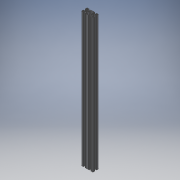
# Autodesk Inventor part: PERFIL_ESTRUTURAL_30X60_640MM
Saved by Autodesk Inventor 2018 (Build 220112000, 112)
## iProperties
Created: 2018-10-10
Part Number: PERFIL_ESTRUTURAL_30X60_640MM
Material: Genérico
Document SubType Name: Modeling
Designer: Georgines
Density: 1 g/cm^3
Appearance: Padrão
Author: Georgines
Autodesk Inventor part; units mm, degrees
ref_plane "YZ Plane" through (0, 0, 0) normal (1, 0, 0) x (0, 1, 0)
ref_plane "XZ Plane" through (0, 0, 0) normal (0, 1, 0) x (-1, 0, 0)
ref_plane "XY Plane" through (0, 0, 0) normal (0, 0, 1) x (1, 0, 0)
sketch "Esboço1" plane through (0, 0, 0) normal (0, 0, 1) x (1, 0, 0)
  arc A0 (-7.8, -13) -> (-7.5, -12.7) centre (-7.8, -12.7) ccw
  line L0 (-10.95, -13) -> (-7.8, -13)
  line L1 (-10.95, -15) -> (-10.95, -13)
  line L2 (-8.4, -15) -> (-10.95, -15)
  line L3 (-8.4, -14.7) -> (-8.4, -15)
  line L4 (-6.2, -14.7) -> (-8.4, -14.7)
  line L5 (-6.2, -15) -> (-6.2, -14.7)
  line L6 (6.2, -15) -> (-6.2, -15)
  line L7 (6.2, -14.7) -> (6.2, -15)
  line L8 (8.4, -14.7) -> (6.2, -14.7)
  line L9 (8.4, -15) -> (8.4, -14.7)
  line L10 (10.95, -15) -> (8.4, -15)
  line L11 (10.95, -13) -> (10.95, -15)
  line L12 (7.8, -13) -> (10.95, -13)
  arc A1 (7.5, -12.7) -> (7.8, -13) centre (7.8, -12.7) ccw
  line L13 (7.5, -11.9376) -> (7.5, -12.7)
  arc A2 (7.5879, -11.7255) -> (7.5, -11.9376) centre (7.8, -11.9376) ccw
  line L14 (10.779, -8.5343) -> (7.5879, -11.7255)
  arc A3 (11.3447, -8.3) -> (10.779, -8.5343) centre (11.3447, -9.1) ccw
  line L15 (18.6553, -8.3) -> (11.3447, -8.3)
  arc A4 (19.221, -8.5343) -> (18.6553, -8.3) centre (18.6553, -9.1) ccw
  line L16 (22.4121, -11.7255) -> (19.221, -8.5343)
  arc A5 (22.5, -11.9376) -> (22.4121, -11.7255) centre (22.2, -11.9376) ccw
  line L17 (22.5, -12.7) -> (22.5, -11.9376)
  arc A6 (22.2, -13) -> (22.5, -12.7) centre (22.2, -12.7) ccw
  line L18 (19.05, -13) -> (22.2, -13)
  line L19 (19.05, -15) -> (19.05, -13)
  line L20 (21.6, -15) -> (19.05, -15)
  line L21 (21.6, -14.7) -> (21.6, -15)
  line L22 (23.8, -14.7) -> (21.6, -14.7)
  line L23 (23.8, -15) -> (23.8, -14.7)
  line L24 (28.5, -15) -> (23.8, -15)
  arc A7 (28.5, -15) -> (30, -13.5) centre (28.5, -13.5) ccw
  line L25 (30, -8.8) -> (30, -13.5)
  line L26 (29.7, -8.8) -> (30, -8.8)
  line L27 (29.7, -6.6) -> (29.7, -8.8)
  line L28 (30, -6.6) -> (29.7, -6.6)
  line L29 (30, -4.05) -> (30, -6.6)
  line L30 (28, -4.05) -> (30, -4.05)
  line L31 (28, -7.2) -> (28, -4.05)
  arc A8 (27.7, -7.5) -> (28, -7.2) centre (27.7, -7.2) ccw
  line L32 (26.9376, -7.5) -> (27.7, -7.5)
  arc A9 (26.7255, -7.4121) -> (26.9376, -7.5) centre (26.9376, -7.2) ccw
  line L33 (23.5343, -4.221) -> (26.7255, -7.4121)
  arc A10 (23.3, -3.6553) -> (23.5343, -4.221) centre (24.1, -3.6553) ccw
  line L34 (23.3, 3.6553) -> (23.3, -3.6553)
  arc A11 (23.5343, 4.221) -> (23.3, 3.6553) centre (24.1, 3.6553) ccw
  line L35 (26.7255, 7.4121) -> (23.5343, 4.221)
  arc A12 (26.9376, 7.5) -> (26.7255, 7.4121) centre (26.9376, 7.2) ccw
  line L36 (27.7, 7.5) -> (26.9376, 7.5)
  arc A13 (28, 7.2) -> (27.7, 7.5) centre (27.7, 7.2) ccw
  line L37 (28, 4.05) -> (28, 7.2)
  line L38 (30, 4.05) -> (28, 4.05)
  line L39 (30, 6.6) -> (30, 4.05)
  line L40 (29.7, 6.6) -> (30, 6.6)
  line L41 (29.7, 8.8) -> (29.7, 6.6)
  line L42 (30, 8.8) -> (29.7, 8.8)
  line L43 (30, 13.5) -> (30, 8.8)
  arc A14 (30, 13.5) -> (28.5, 15) centre (28.5, 13.5) ccw
  line L44 (23.8, 15) -> (28.5, 15)
  line L45 (23.8, 14.7) -> (23.8, 15)
  line L46 (21.6, 14.7) -> (23.8, 14.7)
  line L47 (21.6, 15) -> (21.6, 14.7)
  line L48 (19.05, 15) -> (21.6, 15)
  line L49 (19.05, 13) -> (19.05, 15)
  line L50 (22.2, 13) -> (19.05, 13)
  arc A15 (22.5, 12.7) -> (22.2, 13) centre (22.2, 12.7) ccw
  line L51 (22.5, 11.9376) -> (22.5, 12.7)
  arc A16 (22.4121, 11.7255) -> (22.5, 11.9376) centre (22.2, 11.9376) ccw
  line L52 (19.221, 8.5343) -> (22.4121, 11.7255)
  arc A17 (18.6553, 8.3) -> (19.221, 8.5343) centre (18.6553, 9.1) ccw
  line L53 (11.3447, 8.3) -> (18.6553, 8.3)
  arc A18 (10.779, 8.5343) -> (11.3447, 8.3) centre (11.3447, 9.1) ccw
  line L54 (7.5879, 11.7255) -> (10.779, 8.5343)
  arc A19 (7.5, 11.9376) -> (7.5879, 11.7255) centre (7.8, 11.9376) ccw
  line L55 (7.5, 12.7) -> (7.5, 11.9376)
  arc A20 (7.8, 13) -> (7.5, 12.7) centre (7.8, 12.7) ccw
  line L56 (10.95, 13) -> (7.8, 13)
  line L57 (10.95, 15) -> (10.95, 13)
  line L58 (8.4, 15) -> (10.95, 15)
  line L59 (8.4, 14.7) -> (8.4, 15)
  line L60 (6.2, 14.7) -> (8.4, 14.7)
  line L61 (6.2, 15) -> (6.2, 14.7)
  line L62 (-6.2, 15) -> (6.2, 15)
  line L63 (-6.2, 14.7) -> (-6.2, 15)
  line L64 (-8.4, 14.7) -> (-6.2, 14.7)
  line L65 (-8.4, 15) -> (-8.4, 14.7)
  line L66 (-10.95, 15) -> (-8.4, 15)
  line L67 (-10.95, 13) -> (-10.95, 15)
  line L68 (-7.8, 13) -> (-10.95, 13)
  arc A21 (-7.5, 12.7) -> (-7.8, 13) centre (-7.8, 12.7) ccw
  line L69 (-7.5, 11.9376) -> (-7.5, 12.7)
  arc A22 (-7.5879, 11.7255) -> (-7.5, 11.9376) centre (-7.8, 11.9376) ccw
  line L70 (-10.779, 8.5343) -> (-7.5879, 11.7255)
  arc A23 (-11.3447, 8.3) -> (-10.779, 8.5343) centre (-11.3447, 9.1) ccw
  line L71 (-18.6553, 8.3) -> (-11.3447, 8.3)
  arc A24 (-19.221, 8.5343) -> (-18.6553, 8.3) centre (-18.6553, 9.1) ccw
  line L72 (-22.4121, 11.7255) -> (-19.221, 8.5343)
  arc A25 (-22.5, 11.9376) -> (-22.4121, 11.7255) centre (-22.2, 11.9376) ccw
  line L73 (-22.5, 12.7) -> (-22.5, 11.9376)
  arc A26 (-22.2, 13) -> (-22.5, 12.7) centre (-22.2, 12.7) ccw
  line L74 (-19.05, 13) -> (-22.2, 13)
  line L75 (-19.05, 15) -> (-19.05, 13)
  line L76 (-21.6, 15) -> (-19.05, 15)
  line L77 (-21.6, 14.7) -> (-21.6, 15)
  line L78 (-23.8, 14.7) -> (-21.6, 14.7)
  line L79 (-23.8, 15) -> (-23.8, 14.7)
  line L80 (-28.5, 15) -> (-23.8, 15)
  arc A27 (-28.5, 15) -> (-30, 13.5) centre (-28.5, 13.5) ccw
  line L81 (-30, 8.8) -> (-30, 13.5)
  line L82 (-29.7, 8.8) -> (-30, 8.8)
  line L83 (-29.7, 6.6) -> (-29.7, 8.8)
  line L84 (-30, 6.6) -> (-29.7, 6.6)
  line L85 (-30, 4.05) -> (-30, 6.6)
  line L86 (-28, 4.05) -> (-30, 4.05)
  line L87 (-28, 7.2) -> (-28, 4.05)
  arc A28 (-27.7, 7.5) -> (-28, 7.2) centre (-27.7, 7.2) ccw
  line L88 (-26.9376, 7.5) -> (-27.7, 7.5)
  arc A29 (-26.7255, 7.4121) -> (-26.9376, 7.5) centre (-26.9376, 7.2) ccw
  line L89 (-23.5343, 4.221) -> (-26.7255, 7.4121)
  arc A30 (-23.3, 3.6553) -> (-23.5343, 4.221) centre (-24.1, 3.6553) ccw
  line L90 (-23.3, -3.6553) -> (-23.3, 3.6553)
  arc A31 (-23.5343, -4.221) -> (-23.3, -3.6553) centre (-24.1, -3.6553) ccw
  line L91 (-26.7255, -7.4121) -> (-23.5343, -4.221)
  arc A32 (-26.9376, -7.5) -> (-26.7255, -7.4121) centre (-26.9376, -7.2) ccw
  line L92 (-27.7, -7.5) -> (-26.9376, -7.5)
  arc A33 (-28, -7.2) -> (-27.7, -7.5) centre (-27.7, -7.2) ccw
  line L93 (-28, -4.05) -> (-28, -7.2)
  line L94 (-30, -4.05) -> (-28, -4.05)
  line L95 (-30, -6.6) -> (-30, -4.05)
  line L96 (-29.7, -6.6) -> (-30, -6.6)
  line L97 (-29.7, -8.8) -> (-29.7, -6.6)
  line L98 (-30, -8.8) -> (-29.7, -8.8)
  line L99 (-30, -13.5) -> (-30, -8.8)
  arc A34 (-30, -13.5) -> (-28.5, -15) centre (-28.5, -13.5) ccw
  line L100 (-23.8, -15) -> (-28.5, -15)
  line L101 (-23.8, -14.7) -> (-23.8, -15)
  line L102 (-21.6, -14.7) -> (-23.8, -14.7)
  line L103 (-21.6, -15) -> (-21.6, -14.7)
  line L104 (-19.05, -15) -> (-21.6, -15)
  line L105 (-19.05, -13) -> (-19.05, -15)
  line L106 (-22.2, -13) -> (-19.05, -13)
  arc A35 (-22.5, -12.7) -> (-22.2, -13) centre (-22.2, -12.7) ccw
  line L107 (-22.5, -11.9376) -> (-22.5, -12.7)
  arc A36 (-22.4121, -11.7255) -> (-22.5, -11.9376) centre (-22.2, -11.9376) ccw
  line L108 (-19.221, -8.5343) -> (-22.4121, -11.7255)
  arc A37 (-18.6553, -8.3) -> (-19.221, -8.5343) centre (-18.6553, -9.1) ccw
  line L109 (-11.3447, -8.3) -> (-18.6553, -8.3)
  arc A38 (-10.779, -8.5343) -> (-11.3447, -8.3) centre (-11.3447, -9.1) ccw
  line L110 (-7.5879, -11.7255) -> (-10.779, -8.5343)
  arc A39 (-7.5, -11.9376) -> (-7.5879, -11.7255) centre (-7.8, -11.9376) ccw
  line L111 (-7.5, -12.7) -> (-7.5, -11.9376)
  arc A40 (21.0258, -8.0765) -> (21.0258, -8.5007) centre (21.238, -8.2886) ccw
  line L112 (21.0258, -8.0765) -> (23.0765, -6.0258)
  arc A41 (23.5007, -6.0258) -> (23.0765, -6.0258) centre (23.2886, -6.238) ccw
  line L113 (23.5007, -6.0258) -> (26.187, -8.7121)
  arc A42 (26.187, -8.7121) -> (26.3991, -8.8) centre (26.3991, -8.5) ccw
  line L114 (26.3991, -8.8) -> (28.4, -8.8)
  arc A43 (28.7, -9.1) -> (28.4, -8.8) centre (28.4, -9.1) ccw
  line L115 (28.7, -9.1) -> (28.7, -13.4)
  arc A44 (28.4, -13.7) -> (28.7, -13.4) centre (28.4, -13.4) ccw
  line L116 (28.4, -13.7) -> (24.1, -13.7)
  arc A45 (23.8, -13.4) -> (24.1, -13.7) centre (24.1, -13.4) ccw
  line L117 (23.8, -13.4) -> (23.8, -11.3991)
  arc A46 (23.8, -11.3991) -> (23.7121, -11.187) centre (23.5, -11.3991) ccw
  line L118 (23.7121, -11.187) -> (21.0258, -8.5007)
  arc A47 (9.57, 2.6678) -> (9.5129, 3.0123) centre (9.3007, 2.8001) ccw
  line L119 (9.5129, 3.0123) -> (7.8428, 4.6823)
  arc A48 (7.8428, 5.1066) -> (7.8428, 4.6823) centre (8.0549, 4.8945) ccw
  line L120 (7.8428, 5.1066) -> (9.8934, 7.1572)
  arc A49 (10.3177, 7.1572) -> (9.8934, 7.1572) centre (10.1055, 6.9451) ccw
  line L121 (10.3177, 7.1572) -> (11.9877, 5.4871)
  arc A50 (11.9877, 5.4871) -> (12.3322, 5.43) centre (12.1999, 5.6993) ccw
  arc A51 (13.5232, 5.867) -> (12.3322, 5.43) centre (15, 0) ccw
  arc A52 (13.5232, 5.867) -> (13.75, 6.1579) centre (13.45, 6.1579) ccw
  line L122 (13.75, 6.1579) -> (13.75, 6.7)
  arc A53 (14.05, 7) -> (13.75, 6.7) centre (14.05, 6.7) ccw
  line L123 (14.05, 7) -> (15.95, 7)
  arc A54 (16.25, 6.7) -> (15.95, 7) centre (15.95, 6.7) ccw
  line L124 (16.25, 6.7) -> (16.25, 6.1579)
  arc A55 (16.25, 6.1579) -> (16.4768, 5.867) centre (16.55, 6.1579) ccw
  arc A56 (17.6678, 5.43) -> (16.4768, 5.867) centre (15, 0) ccw
  arc A57 (17.6678, 5.43) -> (18.0123, 5.4871) centre (17.8001, 5.6993) ccw
  line L125 (18.0123, 5.4871) -> (19.6823, 7.1572)
  arc A58 (20.1066, 7.1572) -> (19.6823, 7.1572) centre (19.8945, 6.9451) ccw
  line L126 (20.1066, 7.1572) -> (22.1572, 5.1066)
  arc A59 (22.1572, 4.6823) -> (22.1572, 5.1066) centre (21.9451, 4.8945) ccw
  line L127 (22.1572, 4.6823) -> (20.4871, 3.0123)
  arc A60 (20.4871, 3.0123) -> (20.43, 2.6678) centre (20.6993, 2.8001) ccw
  arc A61 (20.867, 1.4768) -> (20.43, 2.6678) centre (15, 0) ccw
  arc A62 (20.867, 1.4768) -> (21.1579, 1.25) centre (21.1579, 1.55) ccw
  line L128 (21.1579, 1.25) -> (21.7, 1.25)
  arc A63 (22, 0.95) -> (21.7, 1.25) centre (21.7, 0.95) ccw
  line L129 (22, 0.95) -> (22, -0.95)
  arc A64 (21.7, -1.25) -> (22, -0.95) centre (21.7, -0.95) ccw
  line L130 (21.7, -1.25) -> (21.1579, -1.25)
  arc A65 (21.1579, -1.25) -> (20.867, -1.4768) centre (21.1579, -1.55) ccw
  arc A66 (20.43, -2.6678) -> (20.867, -1.4768) centre (15, 0) ccw
  arc A67 (20.43, -2.6678) -> (20.4871, -3.0123) centre (20.6993, -2.8001) ccw
  line L131 (20.4871, -3.0123) -> (22.1572, -4.6823)
  arc A68 (22.1572, -5.1066) -> (22.1572, -4.6823) centre (21.9451, -4.8945) ccw
  line L132 (22.1572, -5.1066) -> (20.1066, -7.1572)
  arc A69 (19.6823, -7.1572) -> (20.1066, -7.1572) centre (19.8945, -6.9451) ccw
  line L133 (19.6823, -7.1572) -> (18.0123, -5.4871)
  arc A70 (18.0123, -5.4871) -> (17.6678, -5.43) centre (17.8001, -5.6993) ccw
  arc A71 (16.4768, -5.867) -> (17.6678, -5.43) centre (15, 0) ccw
  arc A72 (16.4768, -5.867) -> (16.25, -6.1579) centre (16.55, -6.1579) ccw
  line L134 (16.25, -6.1579) -> (16.25, -6.7)
  arc A73 (15.95, -7) -> (16.25, -6.7) centre (15.95, -6.7) ccw
  line L135 (15.95, -7) -> (14.05, -7)
  arc A74 (13.75, -6.7) -> (14.05, -7) centre (14.05, -6.7) ccw
  line L136 (13.75, -6.7) -> (13.75, -6.1579)
  arc A75 (13.75, -6.1579) -> (13.5232, -5.867) centre (13.45, -6.1579) ccw
  arc A76 (12.3322, -5.43) -> (13.5232, -5.867) centre (15, 0) ccw
  arc A77 (12.3322, -5.43) -> (11.9877, -5.4871) centre (12.1999, -5.6993) ccw
  line L137 (11.9877, -5.4871) -> (10.3177, -7.1572)
  arc A78 (9.8934, -7.1572) -> (10.3177, -7.1572) centre (10.1055, -6.9451) ccw
  line L138 (9.8934, -7.1572) -> (7.8428, -5.1066)
  arc A79 (7.8428, -4.6823) -> (7.8428, -5.1066) centre (8.0549, -4.8945) ccw
  line L139 (7.8428, -4.6823) -> (9.5129, -3.0123)
  arc A80 (9.5129, -3.0123) -> (9.57, -2.6678) centre (9.3007, -2.8001) ccw
  arc A81 (9.133, -1.4768) -> (9.57, -2.6678) centre (15, 0) ccw
  arc A82 (9.133, -1.4768) -> (8.8421, -1.25) centre (8.8421, -1.55) ccw
  line L140 (8.8421, -1.25) -> (8.3, -1.25)
  arc A83 (8, -0.95) -> (8.3, -1.25) centre (8.3, -0.95) ccw
  line L141 (8, -0.95) -> (8, 0.95)
  arc A84 (8.3, 1.25) -> (8, 0.95) centre (8.3, 0.95) ccw
  line L142 (8.3, 1.25) -> (8.8421, 1.25)
  arc A85 (8.8421, 1.25) -> (9.133, 1.4768) centre (8.8421, 1.55) ccw
  arc A86 (9.57, 2.6678) -> (9.133, 1.4768) centre (15, 0) ccw
  arc A87 (-9.133, 1.4768) -> (-9.57, 2.6678) centre (-15, 0) ccw
  arc A88 (-9.133, 1.4768) -> (-8.8421, 1.25) centre (-8.8421, 1.55) ccw
  line L143 (-8.8421, 1.25) -> (-8.3, 1.25)
  arc A89 (-8, 0.95) -> (-8.3, 1.25) centre (-8.3, 0.95) ccw
  line L144 (-8, 0.95) -> (-8, -0.95)
  arc A90 (-8.3, -1.25) -> (-8, -0.95) centre (-8.3, -0.95) ccw
  line L145 (-8.3, -1.25) -> (-8.8421, -1.25)
  arc A91 (-8.8421, -1.25) -> (-9.133, -1.4768) centre (-8.8421, -1.55) ccw
  arc A92 (-9.57, -2.6678) -> (-9.133, -1.4768) centre (-15, 0) ccw
  arc A93 (-9.57, -2.6678) -> (-9.5129, -3.0123) centre (-9.3007, -2.8001) ccw
  line L146 (-9.5129, -3.0123) -> (-7.8428, -4.6823)
  arc A94 (-7.8428, -5.1066) -> (-7.8428, -4.6823) centre (-8.0549, -4.8945) ccw
  line L147 (-7.8428, -5.1066) -> (-9.8934, -7.1572)
  arc A95 (-10.3177, -7.1572) -> (-9.8934, -7.1572) centre (-10.1055, -6.9451) ccw
  line L148 (-10.3177, -7.1572) -> (-11.9877, -5.4871)
  arc A96 (-11.9877, -5.4871) -> (-12.3322, -5.43) centre (-12.1999, -5.6993) ccw
  arc A97 (-13.5232, -5.867) -> (-12.3322, -5.43) centre (-15, 0) ccw
  arc A98 (-13.5232, -5.867) -> (-13.75, -6.1579) centre (-13.45, -6.1579) ccw
  line L149 (-13.75, -6.1579) -> (-13.75, -6.7)
  arc A99 (-14.05, -7) -> (-13.75, -6.7) centre (-14.05, -6.7) ccw
  line L150 (-14.05, -7) -> (-15.95, -7)
  arc A100 (-16.25, -6.7) -> (-15.95, -7) centre (-15.95, -6.7) ccw
  line L151 (-16.25, -6.7) -> (-16.25, -6.1579)
  arc A101 (-16.25, -6.1579) -> (-16.4768, -5.867) centre (-16.55, -6.1579) ccw
  arc A102 (-17.6678, -5.43) -> (-16.4768, -5.867) centre (-15, 0) ccw
  arc A103 (-17.6678, -5.43) -> (-18.0123, -5.4871) centre (-17.8001, -5.6993) ccw
  line L152 (-18.0123, -5.4871) -> (-19.6823, -7.1572)
  arc A104 (-20.1066, -7.1572) -> (-19.6823, -7.1572) centre (-19.8945, -6.9451) ccw
  line L153 (-20.1066, -7.1572) -> (-22.1572, -5.1066)
  arc A105 (-22.1572, -4.6823) -> (-22.1572, -5.1066) centre (-21.9451, -4.8945) ccw
  line L154 (-22.1572, -4.6823) -> (-20.4871, -3.0123)
  arc A106 (-20.4871, -3.0123) -> (-20.43, -2.6678) centre (-20.6993, -2.8001) ccw
  arc A107 (-20.867, -1.4768) -> (-20.43, -2.6678) centre (-15, 0) ccw
  arc A108 (-20.867, -1.4768) -> (-21.1579, -1.25) centre (-21.1579, -1.55) ccw
  line L155 (-21.1579, -1.25) -> (-21.7, -1.25)
  arc A109 (-22, -0.95) -> (-21.7, -1.25) centre (-21.7, -0.95) ccw
  line L156 (-22, -0.95) -> (-22, 0.95)
  arc A110 (-21.7, 1.25) -> (-22, 0.95) centre (-21.7, 0.95) ccw
  line L157 (-21.7, 1.25) -> (-21.1579, 1.25)
  arc A111 (-21.1579, 1.25) -> (-20.867, 1.4768) centre (-21.1579, 1.55) ccw
  arc A112 (-20.43, 2.6678) -> (-20.867, 1.4768) centre (-15, 0) ccw
  arc A113 (-20.43, 2.6678) -> (-20.4871, 3.0123) centre (-20.6993, 2.8001) ccw
  line L158 (-20.4871, 3.0123) -> (-22.1572, 4.6823)
  arc A114 (-22.1572, 5.1066) -> (-22.1572, 4.6823) centre (-21.9451, 4.8945) ccw
  line L159 (-22.1572, 5.1066) -> (-20.1066, 7.1572)
  arc A115 (-19.6823, 7.1572) -> (-20.1066, 7.1572) centre (-19.8945, 6.9451) ccw
  line L160 (-19.6823, 7.1572) -> (-18.0123, 5.4871)
  arc A116 (-18.0123, 5.4871) -> (-17.6678, 5.43) centre (-17.8001, 5.6993) ccw
  arc A117 (-16.4768, 5.867) -> (-17.6678, 5.43) centre (-15, 0) ccw
  arc A118 (-16.4768, 5.867) -> (-16.25, 6.1579) centre (-16.55, 6.1579) ccw
  line L161 (-16.25, 6.1579) -> (-16.25, 6.7)
  arc A119 (-15.95, 7) -> (-16.25, 6.7) centre (-15.95, 6.7) ccw
  line L162 (-15.95, 7) -> (-14.05, 7)
  arc A120 (-13.75, 6.7) -> (-14.05, 7) centre (-14.05, 6.7) ccw
  line L163 (-13.75, 6.7) -> (-13.75, 6.1579)
  arc A121 (-13.75, 6.1579) -> (-13.5232, 5.867) centre (-13.45, 6.1579) ccw
  arc A122 (-12.3322, 5.43) -> (-13.5232, 5.867) centre (-15, 0) ccw
  arc A123 (-12.3322, 5.43) -> (-11.9877, 5.4871) centre (-12.1999, 5.6993) ccw
  line L164 (-11.9877, 5.4871) -> (-10.3177, 7.1572)
  arc A124 (-9.8934, 7.1572) -> (-10.3177, 7.1572) centre (-10.1055, 6.9451) ccw
  line L165 (-9.8934, 7.1572) -> (-7.8428, 5.1066)
  arc A125 (-7.8428, 4.6823) -> (-7.8428, 5.1066) centre (-8.0549, 4.8945) ccw
  line L166 (-7.8428, 4.6823) -> (-9.5129, 3.0123)
  arc A126 (-9.5129, 3.0123) -> (-9.57, 2.6678) centre (-9.3007, 2.8001) ccw
  arc A127 (26.3991, 8.8) -> (26.187, 8.7121) centre (26.3991, 8.5) ccw
  line L167 (26.187, 8.7121) -> (23.5007, 6.0258)
  arc A128 (23.0765, 6.0258) -> (23.5007, 6.0258) centre (23.2886, 6.238) ccw
  line L168 (23.0765, 6.0258) -> (21.0258, 8.0765)
  arc A129 (21.0258, 8.5007) -> (21.0258, 8.0765) centre (21.238, 8.2886) ccw
  line L169 (21.0258, 8.5007) -> (23.7121, 11.187)
  arc A130 (23.7121, 11.187) -> (23.8, 11.3991) centre (23.5, 11.3991) ccw
  line L170 (23.8, 11.3991) -> (23.8, 13.4)
  arc A131 (24.1, 13.7) -> (23.8, 13.4) centre (24.1, 13.4) ccw
  line L171 (24.1, 13.7) -> (28.4, 13.7)
  arc A132 (28.7, 13.4) -> (28.4, 13.7) centre (28.4, 13.4) ccw
  line L172 (28.7, 13.4) -> (28.7, 9.1)
  arc A133 (28.4, 8.8) -> (28.7, 9.1) centre (28.4, 9.1) ccw
  line L173 (28.4, 8.8) -> (26.3991, 8.8)
  arc A134 (5.9, -13.7) -> (6.2, -13.4) centre (5.9, -13.4) ccw
  line L174 (5.9, -13.7) -> (-5.9, -13.7)
  arc A135 (-6.2, -13.4) -> (-5.9, -13.7) centre (-5.9, -13.4) ccw
  line L175 (-6.2, -13.4) -> (-6.2, -11.3991)
  arc A136 (-6.2, -11.3991) -> (-6.2879, -11.187) centre (-6.5, -11.3991) ccw
  line L176 (-6.2879, -11.187) -> (-8.9742, -8.5007)
  arc A137 (-8.9742, -8.0765) -> (-8.9742, -8.5007) centre (-8.762, -8.2886) ccw
  line L177 (-8.9742, -8.0765) -> (-6.9235, -6.0258)
  arc A138 (-6.9235, -6.0258) -> (-6.7, -4.0435) centre (-8.0549, -4.8945) ccw
  line L178 (-6.7, -4.0435) -> (-6.7, 4.0435)
  arc A139 (-6.7, 4.0435) -> (-6.9235, 6.0258) centre (-8.0549, 4.8945) ccw
  line L179 (-6.9235, 6.0258) -> (-8.9742, 8.0765)
  arc A140 (-8.9742, 8.5007) -> (-8.9742, 8.0765) centre (-8.762, 8.2886) ccw
  line L180 (-8.9742, 8.5007) -> (-6.2879, 11.187)
  arc A141 (-6.2879, 11.187) -> (-6.2, 11.3991) centre (-6.5, 11.3991) ccw
  line L181 (-6.2, 11.3991) -> (-6.2, 13.4)
  arc A142 (-5.9, 13.7) -> (-6.2, 13.4) centre (-5.9, 13.4) ccw
  line L182 (-5.9, 13.7) -> (5.9, 13.7)
  arc A143 (6.2, 13.4) -> (5.9, 13.7) centre (5.9, 13.4) ccw
  line L183 (6.2, 13.4) -> (6.2, 11.3991)
  arc A144 (6.2, 11.3991) -> (6.2879, 11.187) centre (6.5, 11.3991) ccw
  line L184 (6.2879, 11.187) -> (8.9742, 8.5007)
  arc A145 (8.9742, 8.0765) -> (8.9742, 8.5007) centre (8.762, 8.2886) ccw
  line L185 (8.9742, 8.0765) -> (6.9235, 6.0258)
  arc A146 (6.9235, 6.0258) -> (6.7, 4.0435) centre (8.0549, 4.8945) ccw
  line L186 (6.7, 4.0435) -> (6.7, -4.0435)
  arc A147 (6.7, -4.0435) -> (6.9235, -6.0258) centre (8.0549, -4.8945) ccw
  line L187 (6.9235, -6.0258) -> (8.9742, -8.0765)
  arc A148 (8.9742, -8.5007) -> (8.9742, -8.0765) centre (8.762, -8.2886) ccw
  line L188 (8.9742, -8.5007) -> (6.2879, -11.187)
  arc A149 (6.2879, -11.187) -> (6.2, -11.3991) centre (6.5, -11.3991) ccw
  line L189 (6.2, -11.3991) -> (6.2, -13.4)
  arc A150 (-23.0765, -6.0258) -> (-23.5007, -6.0258) centre (-23.2886, -6.238) ccw
  line L190 (-23.0765, -6.0258) -> (-21.0258, -8.0765)
  arc A151 (-21.0258, -8.5007) -> (-21.0258, -8.0765) centre (-21.238, -8.2886) ccw
  line L191 (-21.0258, -8.5007) -> (-23.7121, -11.187)
  arc A152 (-23.7121, -11.187) -> (-23.8, -11.3991) centre (-23.5, -11.3991) ccw
  line L192 (-23.8, -11.3991) -> (-23.8, -13.4)
  arc A153 (-24.1, -13.7) -> (-23.8, -13.4) centre (-24.1, -13.4) ccw
  line L193 (-24.1, -13.7) -> (-28.4, -13.7)
  arc A154 (-28.7, -13.4) -> (-28.4, -13.7) centre (-28.4, -13.4) ccw
  line L194 (-28.7, -13.4) -> (-28.7, -9.1)
  arc A155 (-28.4, -8.8) -> (-28.7, -9.1) centre (-28.4, -9.1) ccw
  line L195 (-28.4, -8.8) -> (-26.3991, -8.8)
  arc A156 (-26.3991, -8.8) -> (-26.187, -8.7121) centre (-26.3991, -8.5) ccw
  line L196 (-26.187, -8.7121) -> (-23.5007, -6.0258)
  arc A157 (-23.5007, 6.0258) -> (-23.0765, 6.0258) centre (-23.2886, 6.238) ccw
  line L197 (-23.5007, 6.0258) -> (-26.187, 8.7121)
  arc A158 (-26.187, 8.7121) -> (-26.3991, 8.8) centre (-26.3991, 8.5) ccw
  line L198 (-26.3991, 8.8) -> (-28.4, 8.8)
  arc A159 (-28.7, 9.1) -> (-28.4, 8.8) centre (-28.4, 9.1) ccw
  line L199 (-28.7, 9.1) -> (-28.7, 13.4)
  arc A160 (-28.4, 13.7) -> (-28.7, 13.4) centre (-28.4, 13.4) ccw
  line L200 (-28.4, 13.7) -> (-24.1, 13.7)
  arc A161 (-23.8, 13.4) -> (-24.1, 13.7) centre (-24.1, 13.4) ccw
  line L201 (-23.8, 13.4) -> (-23.8, 11.3991)
  arc A162 (-23.8, 11.3991) -> (-23.7121, 11.187) centre (-23.5, 11.3991) ccw
  line L202 (-23.7121, 11.187) -> (-21.0258, 8.5007)
  arc A163 (-21.0258, 8.0765) -> (-21.0258, 8.5007) centre (-21.238, 8.2886) ccw
  line L203 (-21.0258, 8.0765) -> (-23.0765, 6.0258)
  point P0 (0, 0)
  point P1 (0, 0)
  constraints: 408 end point, 328 point on circle, 164 centre point
extrude "Extrusão1" add sketch "Esboço1" along normal blind 700
